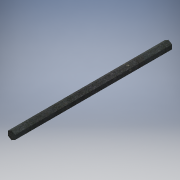
# Autodesk Inventor part: 3-8 hex axle
Saved by Autodesk Inventor 2016 (Build 200138000, 138)
## iProperties
Created: 2016-02-03
Part Number: 3-8 hex axle
Material: Steel
Document SubType Name: Modeling
Designer: gus
Density: 7.85 g/cm^3
Appearance: Plate
Mass: 125.33 g
Surface Area: 68.6184 cm^2
Volume: 15.9656 cm^3
Author: gus
Autodesk Inventor part; units mm, degrees
ref_plane "YZ Plane" through (0, 0, 0) normal (1, 0, 0) x (0, 1, 0)
ref_plane "XZ Plane" through (0, 0, 0) normal (0, 1, 0) x (-1, 0, 0)
ref_plane "XY Plane" through (0, 0, 0) normal (0, 0, 1) x (1, 0, 0)
sketch "Sketch1" plane through (0, 0, 0) normal (0, 0, 1) x (1, 0, 0)
  line L0 (4.7625, -2.7496) -> (0, -5.4993)
  line L1 (0, -5.4993) -> (-4.7625, -2.7496)
  line L2 (-4.7625, -2.7496) -> (-4.7625, 2.7496)
  line L3 (-4.7625, 2.7496) -> (0, 5.4993)
  line L4 (0, 5.4993) -> (4.7625, 2.7496)
  line L5 (4.7625, 2.7496) -> (4.7625, -2.7496)
  point P0 (0, 0)
  point P1 (0, 0)
  dimension "d0" = 9.525
  constraints: 12 end point, 1 coincident, 1 vertical, 13 other
  measures "d0" distance between parallel lines of L5 L2
extrude "Extrusion1" add sketch "Sketch1" along normal blind 203.2
body "Solid1"
